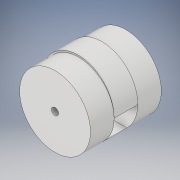
# Autodesk Inventor part: Part2
Saved by Autodesk Inventor 2017 SP1 (Build 210196100, 196)
## iProperties
Created: 2017-05-10
Part Number: Part2
Material: ABS Plastic
Document SubType Name: Modeling
Designer: zallen
Density: 1.06 g/cm^3
Appearance: Smooth - White
Mass: 1957.52 g
Surface Area: 1438.21 cm^2
Volume: 1846.72 cm^3
Author: zallen
Autodesk Inventor part; units mm, degrees
ref_plane "YZ Plane" through (0, 0, 0) normal (1, 0, 0) x (0, 1, 0)
ref_plane "XZ Plane" through (0, 0, 0) normal (0, 1, 0) x (-1, 0, 0)
ref_plane "XY Plane" through (0, 0, 0) normal (0, 0, 1) x (1, 0, 0)
sketch "Sketch1" plane through (0, 0, 0) normal (0, 0, 1) x (1, 0, 0)
  circle A0 centre (0, 0) radius 75
  dimension "d0" = 150
  constraints: 1 centre point, 1 coincident
  measures "d0" diameter of A0
extrude "Extrusion1" add sketch "Sketch1" along normal mid plane 150
sketch "Sketch32" plane through (0, 0, 0) normal (0, 0, 1) x (1, 0, 0)
  line L0 (0, 0) -> (-52, 0)
  line L1 (-52, 0) -> (-52, -75)
  line L2 (-52, -75) -> (0, -75)
  line L3 (0, -75) -> (0, 0)
  dimension "d94" = 52
  dimension "d95" = 75
  constraints: 8 end point, 2 parallel, 1 horizontal, 1 perpendicular
  measures "d94" distance of L2.end L1.end
  measures "d95" distance of L1.end L0.end
extrude "Extrusion23" add sketch "Sketch32" along normal mid plane 75
sketch "Sketch39" plane through (0, 0, -75) normal (0, 0, -1) x (-1, 0, 0)
  circle A0 centre (0, 0) radius 7.5
  dimension "d141" = 15
  constraints: 1 centre point, 1 coincident
  measures "d141" diameter of A0
extrude "Extrusion30" cut sketch "Sketch39" against normal through all
ref_plane "Work Plane4" through (0, 0, 0) normal (0, 0, -1) x (-1, 0, 0)
sketch "Sketch40" plane through (0, 0, 0) normal (0, 0, -1) x (-1, 0, 0)
  circle A0 centre (0, 0) radius 75
  dimension "d144" = 150
  constraints: 1 centre point, 1 coincident
  measures "d144" diameter of A0
extrude "Extrusion31" cut sketch "Sketch40" along normal mid plane 50
sketch "Sketch41" plane through (0, 0, 0) normal (0, 0, -1) x (-1, 0, 0)
  line L0 (52, -75) -> (52, -54.0463) projected
  line L1 (52, -54.0463) -> (-52, -54.0463)
  circle A0 centre (0, 0) radius 75 projected
  arc A1 (-52, -54.0463) -> (0, -75) centre (0, 0) ccw
  constraints: 4 point on circle, 2 end point, 1 centre point, 1 horizontal
extrude "Extrusion32" add sketch "Sketch41" along normal mid plane 50 contours A0 L1 picked at (-14.3807, -56.4807)
sketch "Sketch34" plane through (-52, -75, 37.5) normal (0, -1, 0) x (1, 0, 0)
  circle A0 centre (27, -37.5) radius 25
  line L0 (52, -75) -> (0, -75) projected
  line L1 (-23, -112.5) -> (127, -112.5) projected
  point P0 (52, -37.5)
  dimension "d104" = 50
  dimension "d105" = 25
  dimension "d106" = 37.5
  constraints: 1 centre point
  measures "d104" diameter of A0
  measures "d105" distance of point (52, -37.5) A0.centre
  measures "d106" distance from line of L0 A0.centre
extrude "Extrusion25" cut sketch "Sketch34" against normal blind 10
sketch "Sketch42" plane through (0, 0, 0) normal (0, 0, -1) x (-1, 0, 0)
  arc A0 (52, -54.0463) -> (76.9782, 3.6621) centre (2, 1.8554) ccw
  arc A1 (47, -45.0487) -> (2, 66.8554) centre (2, 1.8554) ccw
  line L0 (47, -45.0487) -> (47, -54.0463)
  line L1 (47, -54.0463) -> (52, -54.0463)
  arc A2 (52, -54.0463) -> (-52, -54.0463) centre (0, 0) ccw projected
  arc A3 (76.9782, 3.6621) -> (-75, 0) centre (0.9891, 1.8311) ccw
  arc A4 (2, 66.8554) -> (-62.9735, 0) centre (2, 1.8554) ccw
  line L2 (-62.9735, 0) -> (-75, 0)
  dimension "d150" = 10
  dimension "d164" = 5
  constraints: 10 point on circle, 6 end point, 4 centre point, 1 horizontal, 1 perpendicular, 1 tangent, 1 vertical
  measures "d150" radial gap between concentric circles of A0 A1
  measures "d164" distance of L0.end L1.end
extrude "Extrusion33" add sketch "Sketch42" along normal mid plane 50
sketch "Sketch43" plane through (52, -54.0463, 25) normal (0, 1, 0) x (1, 0, 0)
  circle A0 centre (-77, 25) radius 25 construction
  line L0 (-62.8579, 10.8579) -> (-91.1421, 10.8579) construction
  line L1 (-91.1421, 10.8579) -> (-91.1421, 39.1421) construction
  line L2 (-91.1421, 39.1421) -> (-62.8579, 39.1421) construction
  line L3 (-62.8579, 39.1421) -> (-62.8579, 10.8579) construction
  line L4 (-62.8579, 10.8579) -> (-91.1421, 39.1421) construction
  line L5 (-91.1421, 10.8579) -> (-62.8579, 39.1421) construction
  circle A1 centre (-91.1421, 39.1421) radius 1.65
  circle A2 centre (-91.1421, 10.8579) radius 1.65
  circle A3 centre (-62.8579, 10.8579) radius 1.65
  circle A4 centre (-62.8579, 39.1421) radius 1.65
  circle A5 centre (-77, 25) radius 3.5
  line L6 (-52, 62.5) -> (-104, 62.5) projected
  line L7 (-52, 25) -> (-52, 62.5) projected
  dimension "d154" = 50
  dimension "d155" = 28.2843
  dimension "d156" = 28.2843
  dimension "d157" = 3.3
  dimension "d158" = 3.3
  dimension "d159" = 3.3
  dimension "d160" = 3.3
  dimension "d163" = 7
  dimension "d165" = 37.5
  dimension "d166" = 25
  constraints: 12 end point, 6 centre point, 5 coincident, 2 midpoint, 2 parallel, 1 horizontal, 1 perpendicular, 1 other
  measures "d154" diameter of A0
  measures "d155" distance of L1.end L2.end
  measures "d156" distance of L0.end L1.end
  measures "d157" diameter of A1
  measures "d158" diameter of A2
  measures "d159" diameter of A3
  measures "d160" diameter of A4
  measures "d163" diameter of A5
  measures "d165" distance from line of L6 A0.centre
  measures "d166" distance from line of L7 A0.centre
extrude "Extrusion34" cut sketch "Sketch43" against normal through all
sketch "Sketch44" plane through (0, 0, -75) normal (0, 0, -1) x (-1, 0, 0)
  arc A0 (75, 0) -> (0, -75) centre (0, 0) ccw construction
  circle A1 centre (0, 0) radius 75 projected
  line L0 (0, 0) -> (107.3838, 0) construction
  arc A2 (50, 0) -> (-50, 0) centre (0, 0) ccw
  arc A3 (40, 0) -> (-40, 0) centre (0, 0) ccw
  line L1 (40, 0) -> (50, 0)
  line L2 (0, -55) -> (0, -55.9017)
  line L3 (-52, -54.0463) -> (47, -54.0463) projected
  line L4 (0, -75) -> (52, -75) projected
  line L5 (-50, 0) -> (-40, 0)
  dimension "d167" = 25
  dimension "d168" = 10
  constraints: 10 point on circle, 8 end point, 3 centre point, 2 horizontal, 1 coincident, 1 collinear, 1 point on line
  measures "d167" radial gap between concentric circles of A0 A2
  measures "d168" radial gap between concentric circles of A2 A3
extrude "Extrusion35" cut sketch "Sketch44" against normal blind 50 contours L1 A3 L5 A2
body "Solid1"
